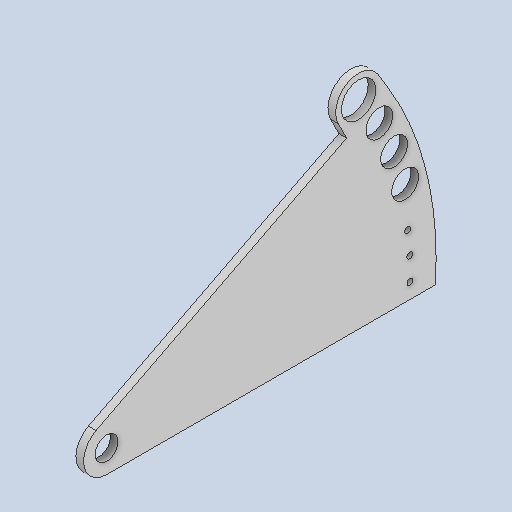
# Autodesk Inventor part: Shooter Side
Saved by Autodesk Inventor 2023 (Build 270158000, 158)
## iProperties
Created: 2023-11-15
Part Number: Shooter Side
Material: Generic
Document SubType Name: Modeling
Designer: jackc
Density: 1 g/cm^3
Appearance: Default
Author: jackc
Autodesk Inventor part; units mm, degrees
ref_plane "YZ Plane" through (0, 0, 0) normal (1, 0, 0) x (0, 1, 0)
ref_plane "XZ Plane" through (0, 0, 0) normal (0, 1, 0) x (-1, 0, 0)
ref_plane "XY Plane" through (0, 0, 0) normal (0, 0, 1) x (1, 0, 0)
sketch "Sketch1" plane through (0, 0, 0) normal (1, 0, 0) x (0, 1, 0)
  circle A0 centre (0, 0) radius 9.525
  arc A1 (-22.7645, -240.2238) -> (126.4053, -205.5417) centre (0, 0) ccw construction
  arc A2 (16.9642, 8.6671) -> (-19.05, 0) centre (0, 0) ccw
  line L0 (-19.05, 0) -> (-19.05, -272.3847)
  circle A3 centre (120.3287, -225.958) radius 14.7 construction
  circle A4 centre (93.6281, -238.2641) radius 14.7 construction
  circle A5 centre (65.6927, -247.4277) radius 14.7 construction
  circle A6 centre (120.3287, -225.958) radius 11.1125
  circle A7 centre (93.6281, -238.2641) radius 11.1125
  circle A8 centre (65.6927, -247.4277) radius 11.1125
  circle A9 centre (120.3287, -225.958) radius 12.7 construction
  circle A10 centre (93.6281, -238.2641) radius 12.7 construction
  circle A11 centre (65.6927, -247.4277) radius 12.7 construction
  line L1 (16.9642, 8.6671) -> (123.0403, -198.9555)
  arc A12 (-19.05, -250.7374) -> (131.0416, -214.6164) centre (0, 0) ccw construction
  arc A13 (-19.05, -272.3847) -> (140.8905, -233.8935) centre (0, 0) ccw
  circle A14 centre (31.658, -249.4592) radius 2.4892
  circle A15 centre (12.6823, -251.14) radius 2.4892
  circle A16 centre (-6.3662, -251.3794) radius 2.4892
  arc A17 (-19.05, -260.9255) -> (135.6769, -223.6891) centre (0, 0) ccw construction
  line L2 (0, 0) -> (7.3253, -241.1888) construction
  line L3 (7.6337, -251.3441) -> (7.9422, -261.4994) construction
  line L4 (7.6337, -251.3441) -> (7.3253, -241.1888) construction
  line L5 (50.997, -247.7827) -> (31.658, -249.4592) construction
  line L6 (48.4264, -236.3907) -> (54.7983, -267.4948) construction
  line L7 (48.4264, -236.3907) -> (0, 0) construction
  circle A18 centre (145.5521, -208.8463) radius 14.2875
  arc A19 (155.3817, -225.1645) -> (136.885, -191.8821) centre (145.5521, -208.8463) ccw
  line L8 (136.885, -191.8821) -> (123.0403, -198.9555)
  line L9 (126.4053, -205.5417) -> (140.8905, -233.8935) construction
  line L10 (123.0403, -198.9555) -> (126.4053, -205.5417) construction
  line L11 (155.3817, -225.1645) -> (140.8905, -233.8935)
  dimension "d0" = 19.05
  dimension "d1" = 241.3
  dimension "d3" = 22.225
  dimension "d4" = 25.4
  dimension "d5" = 2
  dimension "d8" = 9.525
  dimension "d10" = 31.75
  dimension "d11" = 4.9784
  dimension "d12" = 19.05
  dimension "d13" = 19.05
  dimension "d14" = 12.7
  dimension "d17" = 261.62
  dimension "d19" = 19.05
  dimension "d20" = 28.575
  dimension "d22" = 4.7625
  dimension "d24" = 30.48
  constraints: 24 end point, 22 point on circle, 19 centre point, 10 tangent, 8 equal radius, 7 coincident, 6 concentric, 6 point on line, 5 collinear, 2 perpendicular, 1 vertical, 7 other
  measures "d0" diameter of A0
  measures "d1" radius of A1
  measures "d3" diameter of A8
  measures "d4" diameter of A9
  measures "d5" radial gap between concentric circles of A3 A9
  measures "d8" radial gap between concentric circles of A0 A2
  measures "d10" radial gap between concentric circles of A13 A1
  measures "d11" diameter of A16
  measures "d12" distance of A16.centre A15.centre
  measures "d13" distance of A15.centre L5.end
  measures "d14" distance of A12.start A16.centre
  measures "d17" radius of A17
  measures "d19" distance from line of L5.end L6
  measures "d20" diameter of A18
  measures "d22" radial gap between concentric circles of A19 A18
  measures "d24" distance of A18.centre A3.centre
extrude "Extrusion1" add sketch "Sketch1" along normal blind 6.35
equation "\"d1\" = BallSize + 0.5 * WheelSize - Compression"
equation "\"BallSize\" = 203.2"
equation "\"WheelSize\" = 101.6"
equation "\"Compression\" = 12.7"
body "Solid1"
